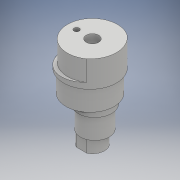
# Autodesk Inventor part: ecc_shaft
Saved by Autodesk Inventor 2017 (Build 210142000, 142)
## iProperties
Created: 2021-02-24
Part Number: ecc_shaft
Material: Generic
Document SubType Name: Modeling
Designer: paulg
Density: 1 g/cm^3
Appearance: Default
Author: paulg
Autodesk Inventor part; units mm, degrees
ref_plane "XZ Plane" through (0, 0, 0) normal (0, 1, 0) x (-1, 0, 0)
ref_plane "XY Plane" through (0, 0, 0) normal (0, 0, 1) x (1, 0, 0)
sketch "Sketch1" plane through (0, 0, 0) normal (0, 0, 1) x (1, 0, 0)
  circle A0 centre (0, 0) radius 2.6
  line L0 (0, 0) -> (-1, 0)
  circle A1 centre (-1, 0) radius 10
  dimension "d0" = 5.2
  dimension "d1" = 1
  dimension "d2" = 20
  constraints: 2 centre point, 2 coincident, 2 end point, 1 horizontal
  measures "d0" diameter of A0
  measures "d1" distance of L0.start L0.end
  measures "d2" diameter of A1
extrude "Extrusion1" add sketch "Sketch1" along normal blind 9
sketch "Sketch2" plane through (-1, 0, 9) normal (0, 0, 1) x (1, 0, 0)
  circle A0 centre (1, 0) radius 2.6 projected
  circle A1 centre (0, 0) radius 10 projected
  circle A2 centre (0, 0) radius 11
  dimension "d5" = 1
  constraints: 1 centre point
  measures "d5" radial gap between concentric circles of A1 A2
extrude "Extrusion2" add sketch "Sketch2" along normal blind 1 contours A1 | A2
sketch "Sketch3" plane through (-1, 0, 0) normal (0, 0, -1) x (-1, 0, 0)
  circle A0 centre (-1, 0) radius 2.6 projected
  line L0 (-1, 0) -> (-2, 0)
  circle A1 centre (-2, 0) radius 7
  dimension "d9" = 14
  dimension "d10" = 1
  constraints: 2 end point, 1 centre point, 1 coincident, 1 horizontal
  measures "d9" diameter of A1
  measures "d10" distance of L0.start L0.end
extrude "Extrusion3" add sketch "Sketch3" along normal blind 3
sketch "Sketch4" plane through (1, 0, -3) normal (0, 0, -1) x (-1, 0, 0)
  circle A0 centre (1, 0) radius 2.6 projected
  circle A1 centre (0, 0) radius 7 construction
  circle A2 centre (0, 0) radius 6
  dimension "d13" = 12
  constraints: 1 centre point, 1 coincident
  measures "d13" diameter of A2
extrude "Extrusion4" add sketch "Sketch4" along normal blind 9
sketch "Sketch5" plane through (0, 0, 0) normal (1, 0, 0) x (0, 1, 0)
  line L0 (0, 0) -> (0, 6.5)
  circle A0 centre (0, 6.5) radius 1.5
  dimension "d16" = 3
  dimension "d17" = 6.5
  constraints: 2 end point, 1 centre point, 1 coincident, 1 vertical
  measures "d16" diameter of A0
  measures "d17" distance of L0.start L0.end
extrude "Extrusion5" cut sketch "Sketch5" against normal through all
ref_plane "Work Plane1" through (-5.5, 0, 0) normal (1, 0, 0) x (0, 1, 0)
sketch "Sketch6" plane through (-5.5, 0, 0) normal (1, 0, 0) x (0, 1, 0)
  line L0 (0, 0) -> (0, 6.7) construction
  line L1 (2.8, 5.0834) -> (0, 3.4668)
  line L2 (0, 3.4668) -> (-2.8, 5.0834)
  line L3 (-2.8, 5.0834) -> (-2.8, 8.3166)
  line L4 (-2.8, 8.3166) -> (0, 9.9332)
  line L5 (0, 9.9332) -> (2.8, 8.3166)
  line L6 (2.8, 8.3166) -> (2.8, 5.0834)
  line L7 (-2.8, 8.3166) -> (-2.8, -3.3824)
  line L8 (-2.8, -3.3824) -> (2.8, -3.3824)
  line L9 (2.8, -3.3824) -> (2.8, 8.3166)
  dimension "d21" = 5.6
  dimension "d22" = 6.7
  constraints: 20 end point, 3 vertical, 2 perpendicular, 1 coincident, 13 other
  measures "d21" distance between parallel lines of L6 L3
  measures "d22" distance of L0.start L0.end
extrude "Extrusion6" cut sketch "Sketch6" against normal blind 3
sketch "Sketch7" plane through (1, 0, -12) normal (0, 0, -1) x (-1, 0, 0)
  circle A0 centre (1, 0) radius 2.6 projected
  arc A1 (0.5, 5.9791) -> (0.5, -5.9791) centre (1, 0) ccw
  circle A2 centre (0, 0) radius 6 construction
  circle A3 centre (0, 0) radius 6 projected
  arc A4 (0.5, -5.9791) -> (0.5, 5.9791) centre (0, 0) ccw
  dimension "d26" = 6
  constraints: 4 point on circle, 2 centre point, 2 coincident, 4 other
  measures "d26" radius of A1
extrude "Extrusion7" [suppressed]
sketch "Sketch8" plane through (1, 0, -13) normal (0, 0, -1) x (-1, 0, 0)
  circle A0 centre (1, 0) radius 2.5 projected
  arc A1 (0.5, -5.9791) -> (0.5, 5.9791) centre (0, 0) ccw projected
  arc A2 (0.5, 5.9791) -> (0.5, -5.9791) centre (1, 0) ccw projected
  circle A3 centre (1, 0) radius 5
  dimension "d29" = 10
  constraints: 1 centre point, 1 coincident
  measures "d29" diameter of A3
extrude "Extrusion8" [suppressed]
sketch "Sketch9" plane through (0, 0, 0) normal (1, 0, 0) x (0, 1, 0)
  line L0 (2.5981, -3) -> (-2.5981, -3) projected
  line L1 (-2.5981, 0) -> (2.5981, 0) projected
  line L2 (-7, -3) -> (-7, 0) construction
  line L3 (-10, 0) -> (10, 0) construction
  line L4 (-7, 0) -> (-7, -3) projected
  line L5 (-7, -2) -> (-6, -1)
  line L6 (-7, 0) -> (-6, 0)
  line L7 (-7, 0) -> (-7, -2)
  line L8 (-6, -1) -> (-6, 0)
  line L9 (2.5981, -3) -> (2.5981, 0) projected
  line L10 (-2.5981, 0) -> (-2.5981, -3) projected
  point P0 (0, 0)
  point P1 (7, -3)
  point P2 (7, 0)
  point P3 (7, 0)
  dimension "d32" = 2
  dimension "d33" = 1
  dimension "d34" = 45
  constraints: 11 end point, 3 perpendicular, 2 point on line
  measures "d32" distance from line of L1 L5.start
  measures "d33" distance between parallel lines of L8 L2
  measures "d34" angle of L2 L5
extrude "Extrusion9" cut sketch "Sketch9" along normal through all both and the other way through all contours L6 L8 L5 L4
mirror "Mirror1" about plane through (0, 0, 0) normal (0, 1, 0) of "Extrusion9"
sketch "Sketch10" plane through (-1, 0, 10) normal (0, 0, 1) x (1, 0, 0)
  circle A0 centre (1, 0) radius 2.6 projected
  circle A1 centre (0, 0) radius 11 projected
  circle A2 centre (0, 0) radius 11 projected
  arc A3 (11, 0) -> (11, 0) centre (1, 0) ccw
  arc A4 (7, 8.4853) -> (7, -8.4853) centre (1, 0) ccw
  line L0 (7, -8.4853) -> (7, 8.4853) construction
  arc A5 (7, -8.4853) -> (7, 8.4853) centre (0, 0) ccw construction
  dimension "d38" = 6
  constraints: 12 point on circle, 3 centre point, 3 coincident, 2 end point
  measures "d38" distance from line of L0 point (1, 0)
extrude "Extrusion10" add sketch "Sketch10" along normal blind 10 contours A1 A4 | A3 picked at (-9.063, 1.631)
sketch "Sketch11" plane through (1, 0, -12) normal (0, 0, -1) x (-1, 0, 0)
  circle A0 centre (1, 0) radius 2.6 projected
  circle A1 centre (0, 0) radius 6 projected
  line L0 (3.1794, -4.5) -> (-1.1794, -4.5)
  line L1 (3.1794, 4.5) -> (-1.1794, 4.5)
  line L2 (0, 0) -> (1, 0)
  arc A2 (3.1794, -4.5) -> (3.1794, 4.5) centre (1, 0) ccw
  arc A3 (-1.1794, 4.5) -> (-1.1794, -4.5) centre (1, 0) ccw
  dimension "d42" = 9
  dimension "d43" = 5
  constraints: 6 end point, 4 point on circle, 2 centre point, 2 horizontal, 1 coincident, 1 concentric, 1 parallel, 1 other
  measures "d42" distance between parallel lines of L1 L0
  measures "d43" radius of A3
extrude "Extrusion11" add sketch "Sketch11" along normal blind 6 contours A2 L0 A3 L1
sketch "Sketch12" plane through (1, 0, -18) normal (0, 0, -1) x (-1, 0, 0)
  circle A0 centre (1, 0) radius 3.05
  dimension "d46" = 6.1
  constraints: 1 centre point, 1 coincident
  measures "d46" diameter of A0
extrude "Extrusion12" cut sketch "Sketch12" against normal blind 2
chamfer "Chamfer1" distance 1.5 angle 45 1 edges at (-10.3923, 0, 10)
sketch "Sketch13" plane through (-1, 0, 0) normal (0, 0, -1) x (-1, 0, 0)
  line L0 (4.5, -2.8) -> (4.5, 0) projected
  line L1 (4.5, -2.8) -> (7.5, -2.8) projected
  line L2 (7.5, -2.8) -> (7.5, 0) projected
  line L3 (4.5, 0) -> (7.5, 0) projected
  line L4 (4.5, 0) -> (4.5, 2.8) projected
  line L5 (4.5, 0) -> (7.5, 0) projected
  line L6 (7.5, 0) -> (7.5, 2.8) projected
  line L7 (4.5, 2.8) -> (7.5, 2.8) projected
  line L8 (4.5, 0) -> (7.5, 0) projected
  circle A0 centre (5.6, 0) radius 1.1
  point P0 (-1, 0)
  dimension "d52" = 2.2
  constraints: 1 horizontal alignment, 1 point on line, 2 other
extrude "Extrusion13" cut sketch "Sketch13" against normal through all contours A0 L3 | L3 A0
body "Solid1"
